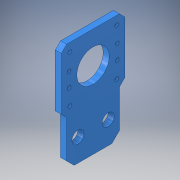
# Autodesk Inventor part: КВ33.044.002 - Деражатель мотора
Saved by Autodesk Inventor 2019 (Build 230136000, 136)
## iProperties
Created: 2019-07-16
Part Number: КВ33.044.002 - Деражатель мотора
Material: Пластик АБС
Document SubType Name: Modeling
Designer: user
Density: 1.06 g/cm^3
Appearance: Голубой
Author: user
Autodesk Inventor part; units mm, degrees
ref_plane "YZ Plane" through (0, 0, 0) normal (1, 0, 0) x (0, 1, 0)
ref_plane "XZ Plane" through (0, 0, 0) normal (0, 1, 0) x (-1, 0, 0)
ref_plane "XY Plane" through (0, 0, 0) normal (0, 0, 1) x (1, 0, 0)
sketch "Эскиз1" plane through (0, 0, 0) normal (1, 0, 0) x (0, 1, 0)
  line L0 (-17.5, 21) -> (-21, 17.5)
  line L1 (-21, 17.5) -> (-21, -17.5)
  line L2 (-21, -17.5) -> (-17.5, -21)
  line L3 (-17.5, -21) -> (17.5, -21)
  line L4 (17.5, -21) -> (21, -17.5)
  line L5 (21, -17.5) -> (21, 17.5)
  line L6 (21, 17.5) -> (17.5, 21)
  line L7 (17.5, 21) -> (-17.5, 21)
  circle A0 centre (0, 0) radius 10.75
  circle A1 centre (-15.5, -15.5) radius 1.25
  circle A2 centre (15.5, -15.5) radius 1.25
  circle A3 centre (15.5, 15.5) radius 1.25
  circle A4 centre (-15.5, 15.5) radius 1.25
  line L8 (-21, 17.5) -> (-51, 17.5)
  line L9 (-51, 17.5) -> (-51, -17.5)
  line L10 (-51, -17.5) -> (-21, -17.5)
  line L11 (-21, -17.5) -> (-21, 17.5)
  line L12 (-51, 0) -> (-36, 0)
  line L13 (-36, 0) -> (-36, 10)
  line L14 (-36, 10) -> (-36, -10)
  circle A5 centre (-36, 10) radius 4
  circle A6 centre (-36, -10) radius 4
  dimension "d0" = 30
  dimension "d1" = 15
  dimension "d2" = 10
  dimension "d3" = 20
  dimension "d4" = 8
  dimension "d5" = 8
  dimension "d12" = 21.5
  constraints: 30 end point, 7 centre point, 2 coincident, 2 horizontal, 2 parallel, 2 perpendicular, 1 midpoint, 1 point on line
  measures "d0" distance of L10.end L9.end
  measures "d1" distance of L12.start L12.end
  measures "d2" distance of L12.end L13.end
  measures "d3" distance of L13.end L14.end
  measures "d4" diameter of A5
  measures "d5" diameter of A6
  measures "d12" diameter of A0
extrude "Выдавливание1" add sketch "Эскиз1" along normal blind 4
chamfer "Фаска1" distance 5 angle 45 2 edges at (2, -51, 17.5) (2, -51, -17.5)
sketch "Эскиз2" plane through (4, 0, 0) normal (1, 0, 0) x (0, 0, -1)
  line L0 (-21, 17.5) -> (-21, -17.5) projected
  line L1 (-21, 0) -> (-16, 0)
  line L2 (-16, 0) -> (-16, 4.75)
  line L3 (-16, 0) -> (-16, -4.75)
  circle A0 centre (-16, 4.75) radius 1.25
  circle A1 centre (-16, -4.75) radius 1.25
  line L4 (21, -17.5) -> (21, 17.5) projected
  line L5 (21, 0) -> (16, 0)
  line L6 (16, 0) -> (16, 4.75)
  line L7 (16, 0) -> (16, -4.75)
  circle A2 centre (16, 4.75) radius 1.25
  circle A3 centre (16, -4.75) radius 1.25
  dimension "d13" = 5
  dimension "d14" = 4.75
  dimension "d15" = 4.75
  dimension "d16" = 2.5
  dimension "d17" = 2.5
  dimension "d18" = 5
  dimension "d19" = 4.75
  dimension "d20" = 4.75
  dimension "d21" = 2.5
  dimension "d22" = 2.5
  constraints: 12 end point, 4 centre point, 4 coincident, 2 horizontal, 2 midpoint, 2 perpendicular, 2 vertical
  measures "d13" distance of L1.start L1.end
  measures "d14" distance of L1.end L2.end
  measures "d15" distance of L1.end L3.end
  measures "d16" diameter of A0
  measures "d17" diameter of A1
  measures "d18" distance of L5.start L5.end
  measures "d19" distance of L5.end L6.end
  measures "d20" distance of L5.end L7.end
  measures "d21" diameter of A2
  measures "d22" diameter of A3
extrude "Выдавливание2" cut sketch "Эскиз2" against normal blind 10
equation "\"d15\" = d14"
equation "\"d17\" = d16"
equation "\"d18\" = d13"
equation "\"d19\" = d14"
equation "\"d20\" = d14"
equation "\"d21\" = d16"
equation "\"d22\" = d16"
